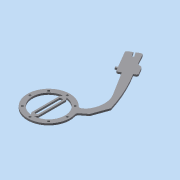
# Autodesk Inventor part: base
Saved by Autodesk Inventor 2015 (Build 190159000, 159)
## iProperties
Created: 2017-10-02
Part Number: base
Material: Generic
Document SubType Name: Modeling
Designer: macbook
Density: 1 g/cm^3
Appearance: Default
Author: macbook
Autodesk Inventor part; units mm, degrees
ref_plane "YZ Plane" through (0, 0, 0) normal (1, 0, 0) x (0, 1, 0)
ref_plane "XZ Plane" through (0, 0, 0) normal (0, 1, 0) x (-1, 0, 0)
ref_plane "XY Plane" through (0, 0, 0) normal (0, 0, 1) x (1, 0, 0)
sketch "Sketch1" plane through (0, 0, 0) normal (0, 0, 1) x (1, 0, 0)
  circle A0 centre (0, 0) radius 65
  dimension "d0" = 130
  constraints: 1 centre point, 1 coincident
  measures "d0" diameter of A0
extrude "Extrusion1" add sketch "Sketch1" along normal blind 5.5
sketch "Sketch5" plane through (0, 0, 5.5) normal (0, 0, 1) x (1, 0, 0)
  line L0 (54.5, 2.75) -> (60, 2.75)
  line L1 (60, 2.75) -> (60, -2.75)
  line L2 (60, -2.75) -> (54.5, -2.75)
  line L3 (54.5, -2.75) -> (54.5, 2.75)
  line L4 (36.5928, 40.4819) -> (40.4819, 44.371)
  line L5 (40.4819, 44.371) -> (44.371, 40.4819)
  line L6 (44.371, 40.4819) -> (40.4819, 36.5928)
  line L7 (40.4819, 36.5928) -> (36.5928, 40.4819)
  line L8 (-2.75, 54.5) -> (-2.75, 60)
  line L9 (-2.75, 60) -> (2.75, 60)
  line L10 (2.75, 60) -> (2.75, 54.5)
  line L11 (2.75, 54.5) -> (-2.75, 54.5)
  line L12 (-40.4819, 36.5928) -> (-44.371, 40.4819)
  line L13 (-44.371, 40.4819) -> (-40.4819, 44.371)
  line L14 (-40.4819, 44.371) -> (-36.5928, 40.4819)
  line L15 (-36.5928, 40.4819) -> (-40.4819, 36.5928)
  line L16 (-54.5, -2.75) -> (-60, -2.75)
  line L17 (-60, -2.75) -> (-60, 2.75)
  line L18 (-60, 2.75) -> (-54.5, 2.75)
  line L19 (-54.5, 2.75) -> (-54.5, -2.75)
  line L20 (-36.5928, -40.4819) -> (-40.4819, -44.371)
  line L21 (-40.4819, -44.371) -> (-44.371, -40.4819)
  line L22 (-44.371, -40.4819) -> (-40.4819, -36.5928)
  line L23 (-40.4819, -36.5928) -> (-36.5928, -40.4819)
  line L24 (2.75, -54.5) -> (2.75, -60)
  line L25 (2.75, -60) -> (-2.75, -60)
  line L26 (-2.75, -60) -> (-2.75, -54.5)
  line L27 (-2.75, -54.5) -> (2.75, -54.5)
  line L28 (40.4819, -36.5928) -> (44.371, -40.4819)
  line L29 (44.371, -40.4819) -> (40.4819, -44.371)
  line L30 (40.4819, -44.371) -> (36.5928, -40.4819)
  line L31 (36.5928, -40.4819) -> (40.4819, -36.5928)
  point P0 (0, 0)
  dimension "d30" = 5.5
  dimension "d31" = 5.5
  dimension "d34" = 360
  constraints: 64 end point, 2 parallel, 1 horizontal, 1 perpendicular, 65 other
  measures "d30" distance of L1.end L2.end
  measures "d31" distance of L0.end L1.end
extrude "Extrusion5" cut sketch "Sketch5" against normal blind 10
sketch "Sketch7" plane through (0, 0, 5.5) normal (0, 0, 1) x (1, 0, 0)
  circle A0 centre (0, 0) radius 65 projected
  line L0 (51.1247, 40.1406) -> (64.8175, 50.8915)
  line L1 (60.6454, 23.3909) -> (84.0046, 41.7313)
  line L2 (84.0046, 41.7313) -> (101.175, 89.1614)
  arc A1 (68.2492, 128.5806) -> (22.61, 201.3724) centre (-8338.3582, -5091.5201) ccw
  arc A2 (101.175, 89.1614) -> (44.4638, 214.134) centre (-401.1925, -63.4539) ccw
  arc A3 (64.8175, 50.8915) -> (68.2492, 128.5806) centre (9.7334, 92.245) ccw
  line L3 (-9.0847, 275.4971) -> (0.0597, 261.7096)
  line L4 (0.0597, 261.7096) -> (-4.5238, 258.6697)
  line L5 (-4.5238, 258.6697) -> (-13.846, 272.7251)
  line L6 (-20.4878, 268.8466) -> (-13.846, 272.7251)
  line L7 (-9.0847, 275.4971) -> (-3.3614, 279.1755)
  line L8 (-20.4878, 268.8466) -> (-29.1232, 263.8039)
  line L9 (-3.3614, 279.1755) -> (5.4134, 283.9717)
  line L10 (11.2184, 194.7202) -> (22.61, 201.3724)
  line L11 (44.4638, 214.134) -> (54.3957, 219.9338)
  line L12 (4.4881, 206.2457) -> (-0.6932, 203.2201)
  line L13 (-0.6932, 203.2201) -> (-3.2145, 207.5378)
  line L14 (-3.2145, 207.5378) -> (1.9667, 210.5634)
  line L15 (-29.1232, 263.8039) -> (1.9667, 210.5634)
  line L16 (4.4881, 206.2457) -> (11.2184, 194.7202)
  line L17 (54.3957, 219.9338) -> (37.2403, 249.3118)
  line L18 (37.2403, 249.3118) -> (27.3211, 243.8901)
  line L19 (27.3211, 243.8901) -> (5.4134, 283.9717)
  dimension "d40" = 250
  dimension "d41" = 20
  dimension "d50" = 5.5
  dimension "d53" = 10
  dimension "d54" = 80
  dimension "d55" = 50
  dimension "d56" = 10
  dimension "d57" = 6
  dimension "d58" = 5
  constraints: 40 end point, 8 perpendicular, 8 point on circle, 3 centre point, 1 line through centre, 1 parallel, 1 tangent
  measures "d40" distance of L1.end L6.start
  measures "d41" distance of L6.start L7.end
  measures "d50" distance between parallel lines of L3 L5
  measures "d53" distance of L6.start L8.end
  measures "d54" distance of L8.end L10.start
  measures "d55" distance of L10.start L11.end
  measures "d56" distance of L7.end L9.end
  measures "d57" distance of L12.start L12.end
  measures "d58" distance of L12.end L13.end
extrude "Extrusion6" add sketch "Sketch7" against normal blind 5.5 contours A0 L0 A3 A1 L10 L16 L12 L13 L14 L15 L8 L6 L5 L4 L3 L7 L9 L19 L18 L17 L11 A2 L2 L1
sketch "Sketch8" plane through (0, 0, 5.5) normal (0, 0, 1) x (1, 0, 0)
  circle A0 centre (0, 0) radius 50
  line L0 (10, 43) -> (10, -43)
  line L1 (-10, -43) -> (-10, 43)
  line L2 (5, 40) -> (-5, 40)
  line L3 (-5, 40) -> (-5, -40)
  line L4 (-5, -40) -> (5, -40)
  line L5 (5, -40) -> (5, 40)
  line L6 (10, -43) -> (5, -49.7494)
  line L7 (-10, -43) -> (-5, -49.7494)
  line L8 (-10, 43) -> (-5, 49.7494)
  line L9 (5, 49.7494) -> (10, 43)
  dimension "d44" = 100
  dimension "d45" = 10
  dimension "d46" = 80
  constraints: 20 end point, 4 parallel, 4 point on circle, 1 centre point, 1 coincident, 1 horizontal, 1 perpendicular, 1 point on line, 1 vertical
  measures "d44" diameter of A0
  measures "d45" distance of L4.end L3.end
  measures "d46" distance of L3.end L2.end
extrude "Extrusion7" cut sketch "Sketch8" against normal blind 5.5 contours A0 L6 L0 L9 | L8 L1 L7 A0 | L5 L4 L3 L2
fillet "Fillet1" radius 3 8 edges at (10, 43, 2.75) (10, -43, 2.75) (-5, 40, 2.75) (-10, -43, 2.75) (5, 40, 2.75) (-10, 43, 2.75) (-5, -40, 2.75) (5, -40, 2.75)
fillet "Fillet2" radius 5 2 edges at (101.175, 89.1614, 2.75) (84.0046, 41.7313, 2.75)
fillet "Fillet3" radius 8 2 edges at (60.6454, 23.3909, 2.75) (51.1247, 40.1406, 2.75)
fillet "Fillet4" radius 5 4 edges at (54.3957, 219.9338, 2.75) (11.2184, 194.7202, 2.75) (5.4134, 283.9717, 2.75) (-29.1232, 263.8039, 2.75)
fillet "Fillet5" radius 8 2 edges at (27.3211, 243.8901, 2.75) (37.2403, 249.3118, 2.75)
body "Solid1"
